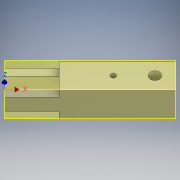
# Autodesk Inventor part: Piston Block
Saved by Autodesk Inventor 2018 (Build 220112000, 112)
## iProperties
Created: 2017-09-20
Part Number: Piston Block
Material: Generic
Document SubType Name: Modeling
Designer: Intel
Density: 1 g/cm^3
Appearance: Stainless - Brushed
Author: Intel
Autodesk Inventor part; units mm, degrees
ref_plane "YZ Plane" through (0, 0, 0) normal (1, 0, 0) x (0, 1, 0)
ref_plane "XZ Plane" through (0, 0, 0) normal (0, 1, 0) x (-1, 0, 0)
ref_plane "XY Plane" through (0, 0, 0) normal (0, 0, 1) x (1, 0, 0)
sketch "Sketch1" plane through (0, 0, 0) normal (0, 0, 1) x (1, 0, 0)
  line L0 (-9.398, -39.6875) -> (9.398, -39.6875)
  line L1 (9.398, -39.6875) -> (9.398, 39.6875)
  line L2 (9.398, 39.6875) -> (-9.398, 39.6875)
  line L3 (-9.398, 39.6875) -> (-9.398, -39.6875)
  line L4 (-9.398, -39.6875) -> (9.398, 39.6875) construction
  line L5 (9.398, -39.6875) -> (-9.398, 39.6875) construction
  point P0 (0, 0)
  dimension "d0" = 18.796
  dimension "d1" = 79.375
  constraints: 12 end point, 2 midpoint, 2 parallel, 1 horizontal, 1 perpendicular
  measures "d0" distance of L2.end L1.end
  measures "d1" distance of L1.end L0.end
extrude "Extrusion1" add sketch "Sketch1" along normal blind 18.796
sketch "Sketch2" plane through (0, 0, 18.796) normal (0, 0, 1) x (1, 0, 0)
  circle A0 centre (0, 30.1625) radius 3.175
  line L0 (9.398, -39.6875) -> (9.398, 39.6875) projected
  line L1 (9.398, 39.6875) -> (-9.398, 39.6875) projected
  point P0 (0, 0)
  dimension "d4" = 6.35
  dimension "d5" = 9.398
  dimension "d6" = 9.525
  constraints: 1 centre point
  measures "d4" diameter of A0
  measures "d5" distance from line of L0 A0.centre
  measures "d6" distance from line of L1 A0.centre
extrude "Extrusion2" cut sketch "Sketch2" against normal blind 18.796
sketch "Sketch3" plane through (0, 0, 18.796) normal (0, 0, 1) x (1, 0, 0)
  circle A0 centre (0, 10.8077) radius 1.5875
  line L0 (9.398, -39.6875) -> (9.398, 39.6875) projected
  line L1 (9.398, 39.6875) -> (-9.398, 39.6875) projected
  point P0 (0, 0)
  dimension "d9" = 3.175
  dimension "d10" = 9.398
  dimension "d11" = 28.8798
  constraints: 1 centre point
  measures "d9" diameter of A0
  measures "d10" distance from line of L0 A0.centre
  measures "d11" distance from line of L1 A0.centre
extrude "Extrusion3" cut sketch "Sketch3" against normal blind 9.398
sketch "Sketch4" plane through (-9.398, -39.6875, 0) normal (0, -1, 0) x (1, 0, 0)
  circle A0 centre (9.398, 9.398) radius 6.35
  line L0 (18.796, 0) -> (18.796, 18.796) projected
  line L1 (0, 0) -> (18.796, 0) projected
  point P0 (9.398, 0)
  dimension "d14" = 12.7
  dimension "d15" = 9.398
  dimension "d16" = 9.398
  constraints: 1 centre point
  measures "d14" diameter of A0
  measures "d15" distance from line of L0 A0.centre
  measures "d16" distance from line of L1 A0.centre
extrude "Extrusion4" cut sketch "Sketch4" against normal blind 53.975
sketch "Sketch5" plane through (9.398, -39.6875, 0) normal (1, 0, 0) x (0, 0, -1)
  line L0 (-18.796, 79.375) -> (-18.796, 0) projected
  line L1 (-18.796, 0) -> (-14.0462, 0)
  line L2 (-14.0462, 0) -> (-14.0462, 25.4)
  line L3 (-14.0462, 25.4) -> (-18.796, 25.4)
  line L4 (-18.796, 25.4) -> (-18.796, 0)
  line L5 (0, 0) -> (-4.7498, 0)
  line L6 (-4.7498, 0) -> (-4.7498, 25.4)
  line L7 (-4.7498, 25.4) -> (0, 25.4)
  line L8 (0, 25.4) -> (0, 0)
  line L9 (0, 79.375) -> (-18.796, 79.375) projected
  line L10 (0, 0) -> (0, 79.375) projected
  point P0 (0, 39.6875)
  dimension "d19" = 53.975
  dimension "d20" = 4.7498
  dimension "d21" = 4.7498
  dimension "d22" = 0
  constraints: 16 end point, 4 parallel, 2 horizontal, 2 perpendicular, 2 point on line
  measures "d19" distance between parallel lines of L9 L3
  measures "d20" distance between parallel lines of L0 L2
  measures "d21" distance between parallel lines of L8 L6
  measures "d22" distance between parallel lines of L10 L8
extrude "Extrusion5" cut sketch "Sketch5" against normal blind 53.975
body "Solid1"
